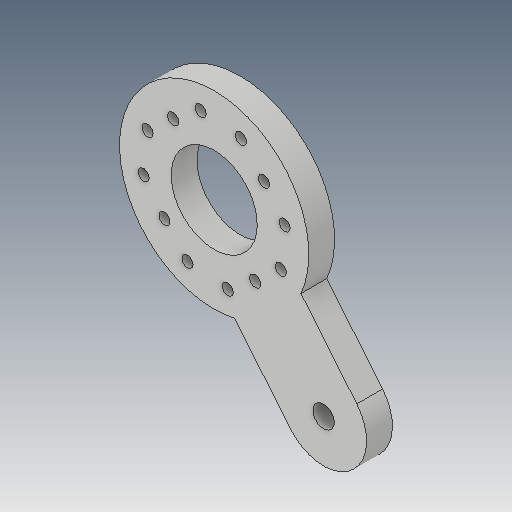
# Autodesk Inventor part: hornLink
Saved by Autodesk Inventor 2019.4 (Build 234330000, 330)
## iProperties
Created: 2018-09-01
Part Number: hornLink
Material: 一般
Document SubType Name: Modeling
Designer: AzLIer
Density: 1 g/cm^3
Appearance: 既定
Author: AzLIer
Autodesk Inventor part; units mm, degrees
note: some values were not read from the file. Chosen so that the rebuilt part matches the saved one: sketch regions of "押し出し1"; arc direction of "押し出し1".
ref_plane "YZ Plane" through (0, 0, 0) normal (1, 0, 0) x (0, 1, 0)
ref_plane "XZ Plane" through (0, 0, 0) normal (0, 1, 0) x (-1, 0, 0)
ref_plane "作業平面1" through (0, 0, 0) normal (0, 0, 1) x (1, 0, 0)
sketch "スケッチ1" plane through (0, 0, 0) normal (0, 0, 1) x (1, 0, 0)
  circle A0 centre (30.9729, -9.6966) radius 0.65 projected
  circle A1 centre (27.8206, 6.7032) radius 0.65 projected
  circle A2 centre (37.1456, -4.6077) radius 0.65 projected
  circle A3 centre (23.6098, -6.2676) radius 0.65 projected
  circle A4 centre (35.1836, 3.2742) radius 0.65 projected
  circle A5 centre (21.6479, 1.6142) radius 0.65 projected
  circle A6 centre (24.6258, 4.2902) radius 0.65 projected
  circle A7 centre (34.1676, -7.2837) radius 0.65 projected
  circle A8 centre (32.5077, 6.2521) radius 0.65 projected
  circle A9 centre (26.2858, -9.2456) radius 0.65 projected
  circle A10 centre (37.5966, 0.0794) radius 0.65 projected
  circle A11 centre (21.1968, -3.0729) radius 0.65 projected
  circle A12 centre (29.3967, -1.4967) radius 1.4 projected
  circle A13 centre (29.3967, -1.4967) radius 10 projected
  circle A14 centre (29.3967, -1.4967) radius 5
  circle A15 centre (42.1192, -16.9285) radius 1.25
  line L0 (29.3967, -1.4967) -> (34.1676, -7.2837)
  circle A16 centre (42.1192, -16.9285) radius 5
  line L1 (38.2612, -20.1091) -> (25.5388, -4.6773)
  line L2 (45.9771, -13.7479) -> (33.2547, 1.6839)
  circle A17 centre (29.3967, -1.4967) radius 11
  point P0 (0, 0)
  dimension "d0" = 10
  dimension "d1" = 2.5
  dimension "d2" = 20
  dimension "d3" = 10
  dimension "d4" = 22
  constraints: 6 end point, 4 centre point, 4 point on circle, 4 tangent, 2 coincident, 1 point on line
  measures "d0" diameter of A14
  measures "d1" diameter of A15
  measures "d2" distance of A12.centre A15.centre
  measures "d3" diameter of A16
  measures "d4" diameter of A17
extrude "押し出し1" add sketch "スケッチ1" along normal blind 3 contours A13 L2 A14 L1 | A13 L1 A17 L2 | L1 A14 L2 A13 | A13 L2 A17 L1 | A17 L2 A16 L1 | A16
